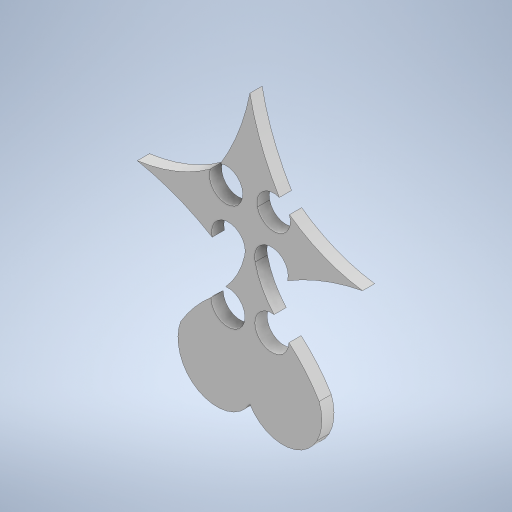
# Autodesk Inventor part: Nobody Emblem
Saved by Autodesk Inventor 2024 (Build 280153000, 153)
## iProperties
Created: 2024-10-02
Part Number: Nobody Emblem
Material: Generic
Document SubType Name: Modeling
Designer: Malik
Density: 1 g/cm^3
Appearance: Default
Author: Malik
Autodesk Inventor part; units mm, degrees
ref_plane "YZ Plane" through (0, 0, 0) normal (1, 0, 0) x (0, 1, 0)
ref_plane "XZ Plane" through (0, 0, 0) normal (0, 1, 0) x (-1, 0, 0)
ref_plane "XY Plane" through (0, 0, 0) normal (0, 0, 1) x (1, 0, 0)
sketch "Sketch1" plane through (0, 0, 0) normal (0, 0, 1) x (1, 0, 0)
  line L0 (-63.3467, 63.7292) -> (61.9288, 63.7292) construction
  line L1 (61.9288, 63.7292) -> (61.9288, -93.0802) construction
  line L2 (61.9288, -93.0802) -> (-63.3467, -93.0802) construction
  line L3 (-63.3467, -93.0802) -> (-63.3467, 63.7292) construction
  line L4 (-0.4255, 162.4475) -> (-0.4255, -218.5525) construction
  line L5 (-278.9224, 0) -> (102.0776, 0) construction
  line L6 (-278.9224, 0) -> (-0.4255, 162.4475) construction
  arc A0 (58.2895, 0.5442) -> (19.2318, -14.4791) centre (81.0298, -116.8596) ccw
  arc A1 (20.1895, 15.8408) -> (58.2895, 0.5442) centre (69.6342, 83.8982) ccw
  arc A2 (3.4987, 10.9772) -> (20.1895, 15.8408) centre (11.9947, 12.8921) ccw
  arc A3 (14.9097, 20.9609) -> (3.4987, 10.9772) centre (11.9125, 12.8736) ccw
  arc A4 (-0.4255, 60.3831) -> (14.9097, 20.9609) centre (117.9773, 83.748) ccw
  arc A5 (-20.0828, -14.4791) -> (-59.1406, 0.5442) centre (-81.8808, -116.8596) ccw
  arc A6 (-59.1406, 0.5442) -> (-21.0406, 15.8408) centre (-70.4853, 83.8982) ccw
  arc A7 (-21.0406, 15.8408) -> (-4.3498, 10.9772) centre (-12.8458, 12.8921) ccw
  arc A8 (-4.3498, 10.9772) -> (-15.7608, 20.9609) centre (-12.7635, 12.8736) ccw
  arc A9 (-15.7608, 20.9609) -> (-0.4255, 60.3831) centre (-118.8283, 83.748) ccw
  arc A10 (-3.1718, -14.4791) -> (-20.0828, -14.4791) centre (-11.6273, -12.1596) ccw
  arc A11 (-20.7493, -42.1086) -> (-13.0628, -33.2545) centre (-11.868, -42.0552) ccw
  arc A12 (-13.0628, -33.2545) -> (-3.1718, -14.4791) centre (-43.3622, -5.2995) ccw
  arc A13 (-35.3697, -79.0918) -> (-0.4255, -80.0922) centre (-17.6172, -69.795) ccw
  arc A14 (-36.5183, -60.7711) -> (-35.3697, -79.0918) centre (-15.4207, -68.6447) ccw
  arc A15 (-20.7493, -42.1086) -> (-36.5183, -60.7711) centre (27.2745, -98.6799) ccw
  arc A16 (19.2318, -14.4791) -> (2.3207, -14.4791) centre (10.7762, -12.1596) ccw
  arc A17 (12.2117, -33.2545) -> (19.8983, -42.1086) centre (11.0169, -42.0552) ccw
  arc A18 (2.3207, -14.4791) -> (12.2117, -33.2545) centre (42.5111, -5.2995) ccw
  arc A19 (-0.4255, -80.0922) -> (34.5187, -79.0918) centre (16.7661, -69.795) ccw
  arc A20 (34.5187, -79.0918) -> (35.6673, -60.7711) centre (14.5697, -68.6447) ccw
  arc A21 (35.6673, -60.7711) -> (19.8983, -42.1086) centre (-28.1255, -98.6799) ccw
  point P0 (0, 0)
  point P1 (-15.8877, 20.9609)
  point P2 (3.8205, 5.0713)
  dimension "d3" = 381
  dimension "d6" = 381
  dimension "d11" = 38.1
  constraints: 44 point on circle, 22 centre point, 21 symmetric about line, 6 end point, 2 point on line, 2 tangent, 1 horizontal, 1 vertical, 13 other
  measures "d3" distance of L4.start L4.end
  measures "d6" distance of L5.start L5.end
  measures "d11" horizontal distance of A0.start A1.start
extrude "Extrusion1" add sketch "Sketch1" against normal blind 6.35
body "Solid1"
